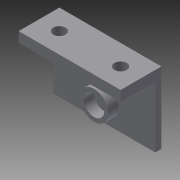
# Autodesk Inventor part: z smooth rod mount
Saved by Autodesk Inventor 2014 SP1 (Build 180222100, 222)
## iProperties
Created: 2014-10-09
Part Number: z smooth rod mount
Material: ABS Plastic
Document SubType Name: Modeling
Designer: Mon
Density: 1.06 g/cm^3
Appearance: Smooth - White
Author: Mon
Autodesk Inventor part; units mm, degrees
ref_plane "YZ Plane" through (0, 0, 0) normal (1, 0, 0) x (0, 1, 0)
ref_plane "XZ Plane" through (0, 0, 0) normal (0, 1, 0) x (-1, 0, 0)
ref_plane "XY Plane" through (0, 0, 0) normal (0, 0, 1) x (1, 0, 0)
sketch "Sketch5" plane through (0, 0, 0) normal (0, 0, 1) x (1, 0, 0)
  line L0 (0, 0) -> (50, 0)
  line L1 (50, 0) -> (50, 20)
  line L2 (50, 20) -> (0, 20)
  line L3 (0, 20) -> (0, 0)
  circle A0 centre (10, 10) radius 3
  circle A1 centre (40, 10) radius 3
  dimension "d43" = 50
  dimension "d44" = 20
  dimension "d47" = 6
  dimension "d48" = 6
  dimension "d49" = 10
  dimension "d50" = 10
  dimension "d51" = 10
  dimension "d52" = 10
  constraints: 8 end point, 2 centre point, 2 parallel, 1 horizontal, 1 perpendicular
  measures "d43" distance of L2.end L1.end
  measures "d44" distance of L1.end L0.end
  measures "d47" diameter of A0
  measures "d48" diameter of A1
  measures "d49" distance from line of L0 A0.centre
  measures "d50" distance from line of L0 A1.centre
  measures "d51" distance from line of L3 A0.centre
  measures "d52" distance from line of L1 A1.centre
extrude "Extrusion5" add sketch "Sketch5" along normal blind 5
sketch "Sketch8" plane through (0, 20, 0) normal (0, 1, 0) x (1, 0, 0)
  line L0 (50, 0) -> (0, 0) projected
  line L1 (0, 0) -> (0, -5) projected
  line L2 (50, -5) -> (0, -5) projected
  line L3 (50, 0) -> (50, -5) projected
  line L4 (0, -5) -> (50, -5)
  line L5 (50, -5) -> (50, 30)
  line L6 (50, 30) -> (0, 30)
  line L7 (0, 30) -> (0, -5)
  line L8 (0, 30) -> (0, 15) construction
  line L9 (0, 0) -> (0, 25) construction
  dimension "d55" = 50
  dimension "d56" = 35
  constraints: 12 end point, 2 parallel, 2 point on line, 1 horizontal, 1 perpendicular
  measures "d55" distance of L6.end L5.end
  measures "d56" distance of L5.end L4.end
extrude "Extrusion6" add sketch "Sketch8" against normal blind 3 contours L0 L7 L6 L5
sketch "Sketch10" plane through (0, 17, 0) normal (0, -1, 0) x (1, 0, 0)
  line L0 (0, 0) -> (50, 0) projected
  line L1 (50, -30) -> (50, 0) projected
  line L2 (25, 0) -> (25, -50.2425) construction
  line L3 (25, 0) -> (25, -20) construction
  line L4 (25, -20) -> (44.8883, -20) construction
  line L5 (44.8883, -20) -> (4.4649, -20) construction
  circle A0 centre (25, -20) radius 5
  circle A1 centre (25, -20) radius 7
  dimension "d68" = 20
  dimension "d69" = 10
  dimension "d70" = 14
  constraints: 8 end point, 2 centre point, 2 coincident, 2 perpendicular, 1 midpoint, 1 parallel, 1 point on line
  measures "d68" distance of L2.start L3.end
  measures "d69" diameter of A0
  measures "d70" diameter of A1
extrude "Extrusion8" add sketch "Sketch10" along normal blind 5
body "Solid2"
